Autodesk Fusion 360 part; units mm, degrees
(part 20 of 20)
  spline S994 degree 3 poles (22.1364, -838.4545) (22.0722, -838.6214) (21.9504, -838.9384) (21.7097, -839.1771) (21.5958, -839.2901) knots 0 0 0 0 0.052961 0.100531 0.100531 0.100531 0.100531
  spline S995 degree 3 poles (21.5958, -839.2901) (21.4642, -839.3761) (21.1885, -839.5562) (20.8591, -839.5752) (20.6869, -839.5851) knots 0 0 0 0 0.046339 0.097057 0.097057 0.097057 0.097057
  spline S996 degree 3 poles (20.6869, -839.5851) (20.4607, -839.5658) (20.0194, -839.5282) (19.7046, -839.2179) (19.5511, -839.0668) knots 0 0 0 0 0.065835 0.128409 0.128409 0.128409 0.128409
  spline S997 degree 3 poles (19.5511, -839.0668) (19.4077, -838.7987) (19.0701, -838.1677) (19.0615, -837.448) (19.0565, -837.034) knots 0 0 0 0 0.090022 0.211899 0.211899 0.211899 0.211899
  line L685 (12.5, 0) -> (12.5, 3)
  line L686 (12.5, 3) -> (27.5, 3)
  line L687 (27.5, 3) -> (27.5, 0)
  line L688 (27.5, 0) -> (12.5, 0)
  spline S998 degree 3 poles (22.5989, -37.0341) (22.5954, -37.3816) (22.5897, -37.949) (22.804, -38.4707) (22.8871, -38.6729) knots 0 0 0 0 0.102785 0.167831 0.167831 0.167831 0.167831
  spline S999 degree 3 poles (22.8871, -38.6729) (22.985, -38.7917) (23.1716, -39.0182) (23.4607, -39.0604) (23.5982, -39.0805) knots 0 0 0 0 0.04439 0.084625 0.084625 0.084625 0.084625
  spline S1000 degree 3 poles (23.5982, -39.0805) (23.7357, -39.0603) (24.0252, -39.0177) (24.2115, -38.7905) (24.3093, -38.6712) knots 0 0 0 0 0.040246 0.084724 0.084724 0.084724 0.084724
  spline S1001 degree 3 poles (24.3093, -38.6712) (24.3924, -38.4689) (24.6064, -37.9476) (24.6009, -37.3809) (24.5975, -37.0341) knots 0 0 0 0 0.065086 0.167658 0.167658 0.167658 0.167658
  spline S1002 degree 3 poles (24.5975, -37.0341) (24.6012, -36.6859) (24.6071, -36.1179) (24.3924, -35.5957) (24.3093, -35.3936) knots 0 0 0 0 0.102998 0.168003 0.168003 0.168003 0.168003
  spline S1003 degree 3 poles (24.3093, -35.3936) (24.2108, -35.2753) (24.0218, -35.0485) (23.7306, -35.0074) (23.5914, -34.9877) knots 0 0 0 0 0.044426 0.085146 0.085146 0.085146 0.085146
  spline S1004 degree 3 poles (23.5914, -34.9877) (23.4571, -35.0033) (23.1857, -35.0347) (23.0066, -35.2414) (22.9161, -35.3458) knots 0 0 0 0 0.039068 0.078965 0.078965 0.078965 0.078965
  spline S1005 degree 3 poles (22.9161, -35.3458) (22.8245, -35.56) (22.5952, -36.096) (22.5975, -36.6822) (22.5989, -37.0341) knots 0 0 0 0 0.069271 0.173342 0.173342 0.173342 0.173342
  spline S1006 degree 3 poles (18.9052, -35.7483) (18.9136, -35.86) (18.9299, -36.0773) (19.0671, -36.2461) (19.1337, -36.3281) knots 0 0 0 0 0.032733 0.063665 0.063665 0.063665 0.063665
  spline S1007 degree 3 poles (19.1337, -36.3281) (19.2176, -36.3937) (19.3917, -36.5299) (19.6127, -36.5453) (19.7271, -36.5532) knots 0 0 0 0 0.03122 0.064779 0.064779 0.064779 0.064779
  spline S1008 degree 3 poles (19.7271, -36.5532) (19.8388, -36.5451) (20.0556, -36.5293) (20.226, -36.395) (20.3087, -36.3298) knots 0 0 0 0 0.032753 0.063582 0.063582 0.063582 0.063582
  spline S1009 degree 3 poles (20.3087, -36.3298) (20.3748, -36.2509) (20.5078, -36.0923) (20.5262, -35.886) (20.5355, -35.7824) knots 0 0 0 0 0.030119 0.060538 0.060538 0.060538 0.060538
  spline S1010 degree 3 poles (20.5355, -35.7824) (20.5261, -35.6746) (20.5074, -35.4609) (20.37, -35.2962) (20.3018, -35.2145) knots 0 0 0 0 0.031624 0.062735 0.062735 0.062735 0.062735
  spline S1011 degree 3 poles (20.3018, -35.2145) (20.2183, -35.1474) (20.0483, -35.0109) (19.8309, -34.9933) (19.7203, -34.9843) knots 0 0 0 0 0.031394 0.063841 0.063841 0.063841 0.063841
  spline S1012 degree 3 poles (19.7203, -34.9843) (19.6091, -34.9928) (19.3919, -35.0093) (19.2207, -35.1438) (19.1371, -35.2094) knots 0 0 0 0 0.032634 0.063783 0.063783 0.063783 0.063783
  spline S1013 degree 3 poles (19.1371, -35.2094) (19.0695, -35.2877) (18.9353, -35.443) (18.9152, -35.6471) (18.9052, -35.7483) knots 0 0 0 0 0.030232 0.059964 0.059964 0.059964 0.059964
  spline S1014 degree 3 poles (18.7074, -38.0573) (18.7128, -38.1446) (18.7238, -38.3214) (18.7955, -38.4835) (18.8318, -38.5655) knots 0 0 0 0 0.026022 0.052693 0.052693 0.052693 0.052693
  spline S1015 degree 3 poles (18.8318, -38.5655) (18.8786, -38.6428) (18.9725, -38.7982) (19.1252, -38.8964) (19.2019, -38.9458) knots 0 0 0 0 0.026723 0.053693 0.053693 0.053693 0.053693
  spline S1016 degree 3 poles (19.2019, -38.9458) (19.2854, -38.9851) (19.453, -39.0639) (19.6379, -39.0749) (19.7305, -39.0805) knots 0 0 0 0 0.027424 0.055001 0.055001 0.055001 0.055001
  spline S1017 degree 3 poles (19.7305, -39.0805) (19.8696, -39.0699) (20.1409, -39.0493) (20.3534, -38.88) (20.457, -38.7974) knots 0 0 0 0 0.040779 0.079588 0.079588 0.079588 0.079588
  spline S1018 degree 3 poles (20.457, -38.7974) (20.5406, -38.6951) (20.7115, -38.4857) (20.7327, -38.2158) (20.7435, -38.0778) knots 0 0 0 0 0.038665 0.079124 0.079124 0.079124 0.079124
  spline S1019 degree 3 poles (20.7435, -38.0778) (20.7322, -37.9374) (20.71, -37.6619) (20.5345, -37.4489) (20.4485, -37.3445) knots 0 0 0 0 0.041167 0.080756 0.080756 0.080756 0.080756
  spline S1020 degree 3 poles (20.4485, -37.3445) (20.3426, -37.2599) (20.1266, -37.0875) (19.8507, -37.0657) (19.7101, -37.0546) knots 0 0 0 0 0.039695 0.080966 0.080966 0.080966 0.080966
  spline S1021 degree 3 poles (19.7101, -37.0546) (19.5729, -37.0655) (19.3037, -37.0871) (19.0946, -37.2575) (18.9921, -37.3411) knots 0 0 0 0 0.040248 0.078949 0.078949 0.078949 0.078949
  spline S1022 degree 3 poles (18.9921, -37.3411) (18.9091, -37.4437) (18.74, -37.6527) (18.7184, -37.9209) (18.7074, -38.0573) knots 0 0 0 0 0.038666 0.078697 0.078697 0.078697 0.078697
  spline S1023 degree 3 poles (22.575, -137.0341) (22.5715, -137.3816) (22.5658, -137.949) (22.7801, -138.4707) (22.8632, -138.6729) knots 0 0 0 0 0.102785 0.167831 0.167831 0.167831 0.167831
  spline S1024 degree 3 poles (22.8632, -138.6729) (22.9611, -138.7917) (23.1477, -139.0182) (23.4369, -139.0604) (23.5743, -139.0805) knots 0 0 0 0 0.04439 0.084625 0.084625 0.084625 0.084625
  spline S1025 degree 3 poles (23.5743, -139.0805) (23.7118, -139.0603) (24.0013, -139.0177) (24.1876, -138.7905) (24.2855, -138.6712) knots 0 0 0 0 0.040246 0.084724 0.084724 0.084724 0.084724
  spline S1026 degree 3 poles (24.2855, -138.6712) (24.3685, -138.4689) (24.5825, -137.9476) (24.577, -137.3809) (24.5737, -137.0341) knots 0 0 0 0 0.065086 0.167658 0.167658 0.167658 0.167658
  spline S1027 degree 3 poles (24.5737, -137.0341) (24.5773, -136.6859) (24.5832, -136.1179) (24.3685, -135.5957) (24.2855, -135.3936) knots 0 0 0 0 0.102998 0.168003 0.168003 0.168003 0.168003
  spline S1028 degree 3 poles (24.2855, -135.3936) (24.1869, -135.2753) (23.9979, -135.0485) (23.7068, -135.0074) (23.5675, -134.9877) knots 0 0 0 0 0.044426 0.085146 0.085146 0.085146 0.085146
  spline S1029 degree 3 poles (23.5675, -134.9877) (23.4332, -135.0033) (23.1618, -135.0347) (22.9827, -135.2414) (22.8922, -135.3458) knots 0 0 0 0 0.039068 0.078965 0.078965 0.078965 0.078965
  spline S1030 degree 3 poles (22.8922, -135.3458) (22.8006, -135.56) (22.5713, -136.096) (22.5736, -136.6822) (22.575, -137.0341) knots 0 0 0 0 0.069271 0.173342 0.173342 0.173342 0.173342
  spline S1031 degree 3 poles (18.7722, -187.8799) (18.7778, -187.9846) (18.7892, -188.1944) (18.8676, -188.3894) (18.9069, -188.487) knots 0 0 0 0 0.031219 0.062565 0.062565 0.062565 0.062565
  spline S1032 degree 3 poles (18.9069, -188.487) (18.955, -188.5771) (19.0485, -188.752) (19.2069, -188.871) (19.2838, -188.9287) knots 0 0 0 0 0.03022 0.058691 0.058691 0.058691 0.058691
  spline S1033 degree 3 poles (19.2838, -188.9287) (19.3646, -188.973) (19.5233, -189.0599) (19.7035, -189.0737) (19.792, -189.0805) knots 0 0 0 0 0.027299 0.05358 0.05358 0.05358 0.05358
  spline S1034 degree 3 poles (19.792, -189.0805) (19.918, -189.0663) (20.1758, -189.0372) (20.3642, -188.8582) (20.4604, -188.7667) knots 0 0 0 0 0.036994 0.075673 0.075673 0.075673 0.075673
  spline S1035 degree 3 poles (20.4604, -188.7667) (20.5419, -188.6473) (20.7168, -188.391) (20.732, -188.0801) (20.7401, -187.9141) knots 0 0 0 0 0.042537 0.091301 0.091301 0.091301 0.091301
  spline S1036 degree 3 poles (20.7401, -187.9141) (20.732, -187.7543) (20.7169, -187.4549) (20.5443, -187.211) (20.4639, -187.0972) knots 0 0 0 0 0.046854 0.087822 0.087822 0.087822 0.087822
  spline S1037 degree 3 poles (20.4639, -187.0972) (20.3652, -187.0102) (20.1661, -186.8345) (19.9015, -186.8108) (19.7681, -186.7988) knots 0 0 0 0 0.038404 0.077492 0.077492 0.077492 0.077492
  spline S1038 degree 3 poles (19.7681, -186.7988) (19.6346, -186.8112) (19.3678, -186.8361) (19.164, -187.0102) (19.0621, -187.0972) knots 0 0 0 0 0.039172 0.078342 0.078342 0.078342 0.078342
  spline S1039 degree 3 poles (19.0621, -187.0972) (18.9776, -187.2076) (18.8011, -187.4381) (18.7821, -187.7286) (18.7722, -187.8799) knots 0 0 0 0 0.040772 0.085151 0.085151 0.085151 0.085151
  spline S1040 degree 3 poles (22.6088, -237.0342) (22.6053, -237.3816) (22.5996, -237.949) (22.8139, -238.4708) (22.897, -238.673) knots 0 0 0 0 0.102785 0.167831 0.167831 0.167831 0.167831
  spline S1041 degree 3 poles (22.897, -238.673) (22.9949, -238.7918) (23.1815, -239.0182) (23.4707, -239.0605) (23.6081, -239.0806) knots 0 0 0 0 0.04439 0.084625 0.084625 0.084625 0.084625
  spline S1042 degree 3 poles (23.6081, -239.0806) (23.7456, -239.0603) (24.0351, -239.0178) (24.2214, -238.7906) (24.3193, -238.6713) knots 0 0 0 0 0.040246 0.084724 0.084724 0.084724 0.084724
  spline S1043 degree 3 poles (24.3193, -238.6713) (24.4023, -238.4689) (24.6163, -237.9477) (24.6108, -237.3809) (24.6075, -237.0342) knots 0 0 0 0 0.065086 0.167658 0.167658 0.167658 0.167658
  spline S1044 degree 3 poles (24.6075, -237.0342) (24.6111, -236.686) (24.617, -236.118) (24.4023, -235.5957) (24.3193, -235.3937) knots 0 0 0 0 0.102998 0.168003 0.168003 0.168003 0.168003
  spline S1045 degree 3 poles (24.3193, -235.3937) (24.2207, -235.2753) (24.0317, -235.0486) (23.7406, -235.0075) (23.6013, -234.9878) knots 0 0 0 0 0.044426 0.085146 0.085146 0.085146 0.085146
  spline S1046 degree 3 poles (23.6013, -234.9878) (23.467, -235.0033) (23.1956, -235.0347) (23.0165, -235.2414) (22.926, -235.3459) knots 0 0 0 0 0.039068 0.078965 0.078965 0.078965 0.078965
  spline S1047 degree 3 poles (22.926, -235.3459) (22.8344, -235.5601) (22.6051, -236.0961) (22.6074, -236.6822) (22.6088, -237.0342) knots 0 0 0 0 0.069271 0.173342 0.173342 0.173342 0.173342
  spline S1048 degree 3 poles (18.7718, -237.88) (18.7775, -237.9847) (18.7888, -238.1945) (18.8673, -238.3894) (18.9066, -238.4871) knots 0 0 0 0 0.031219 0.062565 0.062565 0.062565 0.062565
  spline S1049 degree 3 poles (18.9066, -238.4871) (18.9547, -238.5771) (19.0481, -238.7521) (19.2066, -238.871) (19.2834, -238.9287) knots 0 0 0 0 0.03022 0.058691 0.058691 0.058691 0.058691
  spline S1050 degree 3 poles (19.2834, -238.9287) (19.3643, -238.973) (19.5229, -239.0599) (19.7032, -239.0737) (19.7916, -239.0805) knots 0 0 0 0 0.027299 0.05358 0.05358 0.05358 0.05358
  spline S1051 degree 3 poles (19.7916, -239.0805) (19.9177, -239.0663) (20.1755, -239.0373) (20.3638, -238.8583) (20.4601, -238.7667) knots 0 0 0 0 0.036994 0.075673 0.075673 0.075673 0.075673
  spline S1052 degree 3 poles (20.4601, -238.7667) (20.5416, -238.6473) (20.7164, -238.3911) (20.7317, -238.0802) (20.7398, -237.9141) knots 0 0 0 0 0.042537 0.091301 0.091301 0.091301 0.091301
  spline S1053 degree 3 poles (20.7398, -237.9141) (20.7317, -237.7543) (20.7165, -237.4549) (20.544, -237.211) (20.4635, -237.0972) knots 0 0 0 0 0.046854 0.087822 0.087822 0.087822 0.087822
  spline S1054 degree 3 poles (20.4635, -237.0972) (20.3649, -237.0102) (20.1658, -236.8346) (19.9012, -236.8108) (19.7678, -236.7988) knots 0 0 0 0 0.038404 0.077492 0.077492 0.077492 0.077492
  spline S1055 degree 3 poles (19.7678, -236.7988) (19.6343, -236.8112) (19.3675, -236.8361) (19.1637, -237.0102) (19.0618, -237.0972) knots 0 0 0 0 0.039172 0.078342 0.078342 0.078342 0.078342
  spline S1056 degree 3 poles (19.0618, -237.0972) (18.9772, -237.2076) (18.8007, -237.4382) (18.7817, -237.7286) (18.7718, -237.88) knots 0 0 0 0 0.040772 0.085151 0.085151 0.085151 0.085151
  spline S1057 degree 3 poles (22.5969, -337.034) (22.5934, -337.3815) (22.5877, -337.9488) (22.8021, -338.4706) (22.8851, -338.6728) knots 0 0 0 0 0.102785 0.167831 0.167831 0.167831 0.167831
  spline S1058 degree 3 poles (22.8851, -338.6728) (22.983, -338.7916) (23.1697, -339.018) (23.4588, -339.0603) (23.5963, -339.0803) knots 0 0 0 0 0.04439 0.084625 0.084625 0.084625 0.084625
  spline S1059 degree 3 poles (23.5963, -339.0803) (23.7338, -339.0601) (24.0232, -339.0176) (24.2096, -338.7903) (24.3074, -338.671) knots 0 0 0 0 0.040246 0.084724 0.084724 0.084724 0.084724
  spline S1060 degree 3 poles (24.3074, -338.671) (24.3904, -338.4687) (24.6044, -337.9474) (24.5989, -337.3807) (24.5955, -337.0339) knots 0 0 0 0 0.065086 0.167658 0.167658 0.167658 0.167658
  spline S1061 degree 3 poles (24.5955, -337.0339) (24.5991, -336.6857) (24.605, -336.1177) (24.3903, -335.5955) (24.3073, -335.3934) knots 0 0 0 0 0.102998 0.168003 0.168003 0.168003 0.168003
  spline S1062 degree 3 poles (24.3073, -335.3934) (24.2087, -335.2751) (24.0197, -335.0484) (23.7286, -335.0072) (23.5893, -334.9876) knots 0 0 0 0 0.044426 0.085146 0.085146 0.085146 0.085146
  spline S1063 degree 3 poles (23.5893, -334.9876) (23.455, -335.0031) (23.1836, -335.0345) (23.0045, -335.2413) (22.914, -335.3457) knots 0 0 0 0 0.039068 0.078965 0.078965 0.078965 0.078965
  spline S1064 degree 3 poles (22.914, -335.3457) (22.8224, -335.5599) (22.5931, -336.0959) (22.5955, -336.6821) (22.5969, -337.034) knots 0 0 0 0 0.069271 0.173342 0.173342 0.173342 0.173342
  line L689 (20.1493, -387.7401) -> (20.1493, -385.4856)
  line L690 (20.1493, -385.4856) -> (18.5839, -387.7401)
  line L691 (18.5839, -387.7401) -> (20.1493, -387.7401)
  spline S1065 degree 3 poles (22.7017, -437.0337) (22.6982, -437.3812) (22.6925, -437.9485) (22.9069, -438.4703) (22.99, -438.6725) knots 0 0 0 0 0.102785 0.167831 0.167831 0.167831 0.167831
  spline S1066 degree 3 poles (22.99, -438.6725) (23.0879, -438.7913) (23.2745, -439.0177) (23.5637, -439.0599) (23.7011, -439.08) knots 0 0 0 0 0.04439 0.084625 0.084625 0.084625 0.084625
  spline S1067 degree 3 poles (23.7011, -439.08) (23.8386, -439.0598) (24.1281, -439.0172) (24.3144, -438.79) (24.4122, -438.6707) knots 0 0 0 0 0.040246 0.084724 0.084724 0.084724 0.084724
  spline S1068 degree 3 poles (24.4122, -438.6707) (24.4953, -438.4683) (24.7092, -437.947) (24.7037, -437.3803) (24.7003, -437.0335) knots 0 0 0 0 0.065086 0.167658 0.167658 0.167658 0.167658
  spline S1069 degree 3 poles (24.7003, -437.0335) (24.7039, -436.6853) (24.7097, -436.1173) (24.495, -435.5951) (24.412, -435.393) knots 0 0 0 0 0.102998 0.168003 0.168003 0.168003 0.168003
  spline S1070 degree 3 poles (24.412, -435.393) (24.3134, -435.2747) (24.1244, -435.048) (23.8332, -435.0069) (23.694, -434.9872) knots 0 0 0 0 0.044426 0.085146 0.085146 0.085146 0.085146
  spline S1071 degree 3 poles (23.694, -434.9872) (23.5597, -435.0028) (23.2883, -435.0342) (23.1092, -435.2409) (23.0187, -435.3454) knots 0 0 0 0 0.039068 0.078965 0.078965 0.078965 0.078965
  spline S1072 degree 3 poles (23.0187, -435.3454) (22.9271, -435.5596) (22.6979, -436.0956) (22.7002, -436.6818) (22.7017, -437.0337) knots 0 0 0 0 0.069271 0.173342 0.173342 0.173342 0.173342
  line L692 (20.154, -437.7399) -> (20.1538, -435.4855)
  line L693 (20.1538, -435.4855) -> (18.5885, -437.74)
  line L694 (18.5885, -437.74) -> (20.154, -437.7399)
  spline S1073 degree 3 poles (22.6014, -537.0337) (22.5979, -537.3811) (22.5923, -537.9485) (22.8067, -538.4702) (22.8897, -538.6724) knots 0 0 0 0 0.102785 0.167831 0.167831 0.167831 0.167831
  spline S1074 degree 3 poles (22.8897, -538.6724) (22.9876, -538.7912) (23.1743, -539.0177) (23.4634, -539.0599) (23.6009, -539.08) knots 0 0 0 0 0.04439 0.084625 0.084625 0.084625 0.084625
  spline S1075 degree 3 poles (23.6009, -539.08) (23.7384, -539.0597) (24.0279, -539.0171) (24.2142, -538.7899) (24.312, -538.6706) knots 0 0 0 0 0.040246 0.084724 0.084724 0.084724 0.084724
  spline S1076 degree 3 poles (24.312, -538.6706) (24.395, -538.4683) (24.609, -537.947) (24.6034, -537.3802) (24.6, -537.0335) knots 0 0 0 0 0.065086 0.167658 0.167658 0.167658 0.167658
  spline S1077 degree 3 poles (24.6, -537.0335) (24.6036, -536.6853) (24.6095, -536.1173) (24.3948, -535.5951) (24.3117, -535.393) knots 0 0 0 0 0.102998 0.168003 0.168003 0.168003 0.168003
  spline S1078 degree 3 poles (24.3117, -535.393) (24.2131, -535.2747) (24.0241, -535.048) (23.733, -535.0068) (23.5937, -534.9872) knots 0 0 0 0 0.044426 0.085146 0.085146 0.085146 0.085146
  spline S1079 degree 3 poles (23.5937, -534.9872) (23.4594, -535.0027) (23.188, -535.0342) (23.0089, -535.2409) (22.9184, -535.3454) knots 0 0 0 0 0.039068 0.078965 0.078965 0.078965 0.078965
  spline S1080 degree 3 poles (22.9184, -535.3454) (22.8268, -535.5596) (22.5976, -536.0956) (22.6, -536.6817) (22.6014, -537.0337) knots 0 0 0 0 0.069271 0.173342 0.173342 0.173342 0.173342
  spline S1081 degree 3 poles (22.641, -637.0339) (22.6375, -637.3814) (22.6319, -637.9488) (22.8462, -638.4705) (22.9293, -638.6728) knots 0 0 0 0 0.102785 0.167831 0.167831 0.167831 0.167831
  spline S1082 degree 3 poles (22.9293, -638.6728) (23.0272, -638.7915) (23.2138, -639.018) (23.5029, -639.0602) (23.6404, -639.0803) knots 0 0 0 0 0.04439 0.084625 0.084625 0.084625 0.084625
  spline S1083 degree 3 poles (23.6404, -639.0803) (23.7779, -639.0601) (24.0674, -639.0175) (24.2537, -638.7903) (24.3515, -638.671) knots 0 0 0 0 0.040246 0.084724 0.084724 0.084724 0.084724
  spline S1084 degree 3 poles (24.3515, -638.671) (24.4346, -638.4687) (24.6486, -637.9474) (24.643, -637.3806) (24.6397, -637.0339) knots 0 0 0 0 0.065086 0.167658 0.167658 0.167658 0.167658
  spline S1085 degree 3 poles (24.6397, -637.0339) (24.6433, -636.6857) (24.6492, -636.1177) (24.4345, -635.5955) (24.3514, -635.3934) knots 0 0 0 0 0.102998 0.168003 0.168003 0.168003 0.168003
  spline S1086 degree 3 poles (24.3514, -635.3934) (24.2528, -635.2751) (24.0639, -635.0483) (23.7727, -635.0072) (23.6335, -634.9875) knots 0 0 0 0 0.044426 0.085146 0.085146 0.085146 0.085146
  spline S1087 degree 3 poles (23.6335, -634.9875) (23.4992, -635.0031) (23.2277, -635.0345) (23.0487, -635.2412) (22.9582, -635.3457) knots 0 0 0 0 0.039068 0.078965 0.078965 0.078965 0.078965
  spline S1088 degree 3 poles (22.9582, -635.3457) (22.8666, -635.5599) (22.6373, -636.0959) (22.6396, -636.682) (22.641, -637.0339) knots 0 0 0 0 0.069271 0.173342 0.173342 0.173342 0.173342
  spline S1089 degree 3 poles (22.363, -737.034) (22.3595, -737.3815) (22.3539, -737.9488) (22.5682, -738.4706) (22.6513, -738.6728) knots 0 0 0 0 0.102785 0.167831 0.167831 0.167831 0.167831
  spline S1090 degree 3 poles (22.6513, -738.6728) (22.7492, -738.7916) (22.9358, -739.018) (23.2249, -739.0603) (23.3624, -739.0803) knots 0 0 0 0 0.04439 0.084625 0.084625 0.084625 0.084625
  spline S1091 degree 3 poles (23.3624, -739.0803) (23.4999, -739.0601) (23.7894, -739.0175) (23.9757, -738.7903) (24.0735, -738.671) knots 0 0 0 0 0.040246 0.084724 0.084724 0.084724 0.084724
  spline S1092 degree 3 poles (24.0735, -738.671) (24.1566, -738.4687) (24.3706, -737.9474) (24.365, -737.3807) (24.3617, -737.0339) knots 0 0 0 0 0.065086 0.167658 0.167658 0.167658 0.167658
  spline S1093 degree 3 poles (24.3617, -737.0339) (24.3653, -736.6857) (24.3712, -736.1177) (24.1565, -735.5955) (24.0734, -735.3934) knots 0 0 0 0 0.102998 0.168003 0.168003 0.168003 0.168003
  spline S1094 degree 3 poles (24.0734, -735.3934) (23.9748, -735.2751) (23.7859, -735.0484) (23.4947, -735.0072) (23.3555, -734.9876) knots 0 0 0 0 0.044426 0.085146 0.085146 0.085146 0.085146
  spline S1095 degree 3 poles (23.3555, -734.9876) (23.2212, -735.0031) (22.9497, -735.0345) (22.7707, -735.2412) (22.6802, -735.3457) knots 0 0 0 0 0.039068 0.078965 0.078965 0.078965 0.078965
  spline S1096 degree 3 poles (22.6802, -735.3457) (22.5886, -735.5599) (22.3593, -736.0959) (22.3616, -736.682) (22.363, -737.034) knots 0 0 0 0 0.069271 0.173342 0.173342 0.173342 0.173342
  spline S1097 degree 3 poles (19.6875, -837.034) (19.684, -837.3815) (19.6783, -837.9489) (19.8927, -838.4706) (19.9758, -838.6728) knots 0 0 0 0 0.102785 0.167831 0.167831 0.167831 0.167831
  spline S1098 degree 3 poles (19.9758, -838.6728) (20.0736, -838.7916) (20.2603, -839.0181) (20.5494, -839.0603) (20.6869, -839.0804) knots 0 0 0 0 0.04439 0.084625 0.084625 0.084625 0.084625
  spline S1099 degree 3 poles (20.6869, -839.0804) (20.8244, -839.0601) (21.1139, -839.0176) (21.3002, -838.7903) (21.398, -838.6711) knots 0 0 0 0 0.040246 0.084724 0.084724 0.084724 0.084724
  spline S1100 degree 3 poles (21.398, -838.6711) (21.4811, -838.4687) (21.695, -837.9474) (21.6895, -837.3807) (21.6861, -837.0339) knots 0 0 0 0 0.065086 0.167658 0.167658 0.167658 0.167658
  spline S1101 degree 3 poles (21.6861, -837.0339) (21.6897, -836.6857) (21.6956, -836.1177) (21.4809, -835.5955) (21.3979, -835.3934) knots 0 0 0 0 0.102998 0.168003 0.168003 0.168003 0.168003
  spline S1102 degree 3 poles (21.3979, -835.3934) (21.2993, -835.2751) (21.1103, -835.0484) (20.8192, -835.0073) (20.6799, -834.9876) knots 0 0 0 0 0.044426 0.085146 0.085146 0.085146 0.085146
  spline S1103 degree 3 poles (20.6799, -834.9876) (20.5456, -835.0031) (20.2742, -835.0346) (20.0951, -835.2413) (20.0046, -835.3457) knots 0 0 0 0 0.039068 0.078965 0.078965 0.078965 0.078965
  spline S1104 degree 3 poles (20.0046, -835.3457) (19.913, -835.5599) (19.6837, -836.0959) (19.6861, -836.6821) (19.6875, -837.034) knots 0 0 0 0 0.069271 0.173342 0.173342 0.173342 0.173342
  line L695 (0, -3) -> (0, -870.7)
  constraint coincident L1.end L2.start
  constraint coincident L326.end L327.start
equation "d94 = '5 cm'"
equation "d104 = '10cm'"
equation "d114 = '15cm'"
equation "d124 = '20cm'"
equation "d134 = '25cm'"
equation "d144 = '30cm'"
equation "d154 = '35cm'"
equation "d164 = '40cm'"
equation "d174 = '45cm'"
equation "d184 = '50cm'"
equation "d194 = '55cm'"
equation "d204 = '60cm'"
equation "d214 = '65cm'"
equation "d224 = '70cm'"
equation "d234 = '75cm'"
equation "d244 = '80cm'"
equation "d246 = '0 cm'"
